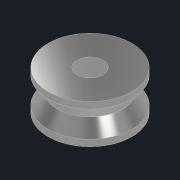
# Autodesk Inventor part: Rope Bearing Pulley
Saved by Autodesk Inventor 2021.3 (Build 253353000, 353)
## iProperties
Created: 2022-07-30
Part Number: Rope Bearing Pulley
Material: Stainless Steel
Document SubType Name: Modeling
Designer: david
Density: 8 g/cm^3
Appearance: Semi-Polished
Author: david
Autodesk Inventor part; units mm, degrees
ref_plane "YZ Plane" through (0, 0, 0) normal (1, 0, 0) x (0, 1, 0)
ref_plane "XZ Plane" through (0, 0, 0) normal (0, 1, 0) x (-1, 0, 0)
ref_plane "XY Plane" through (0, 0, 0) normal (0, 0, 1) x (1, 0, 0)
sketch "Sketch1" plane through (0, 0, 0) normal (0, 0, 1) x (1, 0, 0)
  line L0 (2, -3.03) -> (2, 3.03)
  line L1 (2, -3.03) -> (6.5, -3.03)
  line L2 (2, 3.03) -> (6.5, 3.03)
  line L3 (6.5, 3.03) -> (6.5, 2.03)
  line L4 (0, 0) -> (0.6672, 0) construction
  line L5 (6.5, 2.03) -> (5.1, 0)
  line L6 (6.5, -3.03) -> (6.5, -2.03)
  line L7 (6.5, -2.03) -> (5.1, 0)
  line L8 (0, -4.242) -> (0, 4.242) projected
  dimension "d0" = 2
  dimension "d1" = 6.06
  dimension "d2" = 3.03
  dimension "d3" = 4.5
  dimension "d5" = 1
  dimension "d6" = 5.1
  constraints: 16 end point, 3 horizontal, 2 vertical, 1 symmetric about line
  measures "d0" distance from line of L4.start L0
  measures "d1" distance of L0.start L0.end
  measures "d2" vertical distance of L4.start L0.start
  measures "d3" distance of L0.start L1.end
  measures "d5" distance of L2.end L3.end
  measures "d6" distance of L4.start L5.end
revolve "Revolution1" add sketch "Sketch1" angle 360 about axis through (0, -10, 0) along (0, 1, 0)
equation "\"d2\" = 0.5 * d1"
body "Solid1"
